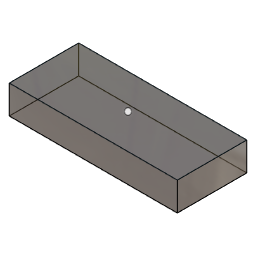
Base Assembly FINAL v1 (Autodesk Fusion 360 archive; units mm, degrees)
design "Stock base"
Autodesk Fusion 360 part; units mm, degrees
sketch "Sketch1" plane through (0, 0, 0) normal (0, 0, 1) x (1, 0, 0)
  line L0 (0, 0) -> (93.472, 0)
  line L1 (93.472, 0) -> (93.472, 38.608)
  line L2 (93.472, 38.608) -> (0, 38.608)
  line L3 (0, 38.608) -> (0, 0)
  dimension "d1" = 93.472
  dimension "d2" = 38.608
  constraint horizontal L0
  constraint vertical L1
  constraint horizontal L2
  constraint vertical L3
  constraint coincident L0.start L3.end
  measures "d1" distance of L1.end L2.end
  measures "d2" distance of L0.start L2.end
extrude "Extrude1" add sketch "Sketch1" along normal blind 15.875
sketch "Sketch2" plane through (0, 0, 15.875) normal (0, 0, 1) x (-1, 0, 0)
  line L0 (0, -38.608) -> (0, 0)
  line L1 (0, 0) -> (-93.472, 0)
  line L2 (-93.472, 0) -> (-93.472, -38.608)
  line L3 (-93.472, -38.608) -> (0, -38.608)
  point P0 (-46.736, -19.304)
  dimension "d8" = 38.608
  dimension "d9" = 93.472
  dimension "d10" = 46.736
  dimension "d11" = 19.304
  measures "d8" distance of L1.end L2.end
  measures "d9" distance of L0.start L2.end
  measures "d10" distance of L2 P0
  measures "d11" distance of L1 P0
equation "d10 = d9 / 2"
equation "d11 = d8 / 2"
